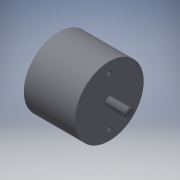
# Autodesk Inventor part: Motor50
Saved by Autodesk Inventor 2018 (Build 220112000, 112)
## iProperties
Created: 2013-02-18
Part Number: Motor50
Material: Steel
Document SubType Name: Modeling
Designer: Neef
Density: 7.85 g/cm^3
Mass: 573.284 g
Surface Area: 103.73 cm^2
Volume: 73.0298 cm^3
Appearance: Steel
Author: Neef
Autodesk Inventor part; units mm, degrees
ref_plane "YZ Plane" through (0, 0, 0) normal (1, 0, 0) x (0, 1, 0)
ref_plane "XZ Plane" through (0, 0, 0) normal (0, 1, 0) x (-1, 0, 0)
ref_plane "XY Plane" through (0, 0, 0) normal (0, 0, 1) x (1, 0, 0)
sketch "Skizze1" plane through (0, 0, 0) normal (0, 0, 1) x (1, 0, 0)
  line L0 (0, 30) -> (0, -5) projected
  line L1 (-17.6, 0) -> (63.6, 0) projected
  line L2 (-6, 0) -> (-6, 3)
  line L3 (-6, 3) -> (0, 3)
  line L4 (0, 3) -> (0, 25)
  line L5 (0, 25) -> (37, 25)
  line L6 (37, 25) -> (37, 3)
  line L7 (37, 3) -> (52, 3)
  line L8 (52, 3) -> (52, 0)
  point P0 (0, 0)
  dimension "d0" = 15
  dimension "d2" = 37
  dimension "d3" = 58
  dimension "d4" = 25
  dimension "d5" = 3
  dimension "d6" = 3
  constraints: 14 end point, 5 perpendicular, 4 point on line, 1 parallel
  measures "d0" distance of L6.end L7.end
  measures "d2" distance of L4.end L5.end
  measures "d3" distance between parallel lines of L2 L8
  measures "d4" distance between parallel lines of L1 L5
  measures "d5" distance between parallel lines of L1 L3
  measures "d6" distance between parallel lines of L1 L7
revolve "Umdrehung1" add sketch "Skizze1" angle 360 about axis through (0, 0, 0) along (1, 0, 0)
sketch "Skizze2" plane through (37, 0, 0) normal (1, 0, 0) x (0, 0, -1)
  circle A0 centre (0, 0) radius 3 projected
  point P0 (-17.5, 0)
  point P1 (17.5, 0)
  dimension "d8" = 35
  dimension "d9" = 17.5
  measures "d8" distance of point (17.5, 0) point (-17.5, 0)
  measures "d9" distance of A0.centre point (-17.5, 0)
hole "Bohrung1" at (37, 0, 17.5) at (37, 0, -17.5) direction (-1, 0, 0) diameter 3.242 depth 6 tip angle 118 thread size "M4x0.7" class "6H" standard "ISO Metric profile"
chamfer "Fase1" distance 0.5 angle 45 2 edges at (52, -3, 0) (-6, -3, 0)
equation "\"d9\" = 0.5 * d8"
equation "\"d6\" = d5"
